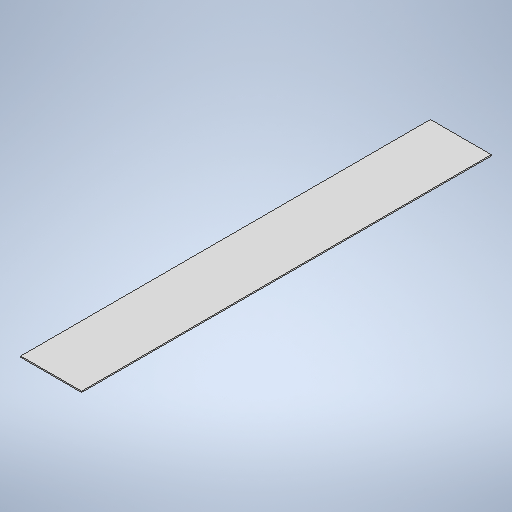
# Autodesk Inventor part: 가로로만 윗판
Saved by Autodesk Inventor 2025.1 (Build 291241000, 241)
## iProperties
Created: 2024-10-29
Part Number: 가로로만 윗판
Material: 일반
Document SubType Name: Modeling
Designer: gmsee
Density: 1 g/cm^3
Appearance: 기본값
Author: gmsee
Autodesk Inventor part; units mm, degrees
ref_plane "YZ Plane" through (0, 0, 0) normal (1, 0, 0) x (0, 1, 0)
ref_plane "XZ Plane" through (0, 0, 0) normal (0, 1, 0) x (-1, 0, 0)
ref_plane "XY Plane" through (0, 0, 0) normal (0, 0, 1) x (1, 0, 0)
sketch "스케치1" plane through (0, 0, 0) normal (0, 1, 0) x (-1, 0, 0)
  line L0 (52, 350) -> (-52, 350)
  line L1 (-52, 350) -> (-52, -350)
  line L2 (-52, -350) -> (52, -350)
  line L3 (52, -350) -> (52, 350)
  point P0 (0, 0)
  dimension "d0" = 700
  dimension "d1" = 350
  dimension "d2" = 104
  dimension "d3" = 52
  constraints: 8 end point, 2 parallel, 1 horizontal, 1 perpendicular
  measures "d0" distance of L2.end L0.start
  measures "d1" distance from line of L2 point (0, 0)
  measures "d2" distance between parallel lines of L1 L3
  measures "d3" distance from line of L1 point (0, 0)
extrude "돌출1" add sketch "스케치1" along normal blind 2
equation "\"d1\" = 0.5 * d0"
equation "\"d3\" = 0.5 * d2"
